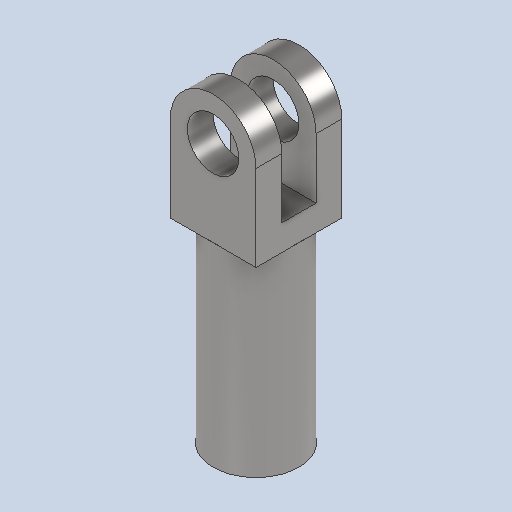
# Autodesk Inventor part: Część L5
Saved by Autodesk Inventor 2022.1 (Build 261234020, 234B)
## iProperties
Created: 2022-05-02
Part Number: Część L5
Material: Stal nierdzewna 440C
Document SubType Name: Modeling
Designer: Kacper Kaczmarski
Density: 7.75 g/cm^3
Appearance: Częściowo polerowany
Mass: 19.5633 g
Surface Area: 16.5661 cm^2
Volume: 2.5243 cm^3
Author: Kacper Kaczmarski
Autodesk Inventor part; units mm, degrees
ref_plane "YZ Plane" through (0, 0, 0) normal (1, 0, 0) x (0, 1, 0)
ref_plane "XZ Plane" through (0, 0, 0) normal (0, 1, 0) x (-1, 0, 0)
ref_plane "XY Plane" through (0, 0, 0) normal (0, 0, 1) x (1, 0, 0)
sketch "Szkic1" plane through (0, 0, 0) normal (0, 0, 1) x (1, 0, 0)
  line L0 (0, 0) -> (-10, 0)
  line L1 (-10, 0) -> (-10, 32.68)
  line L2 (-10, 32.68) -> (0, 32.68)
  line L3 (0, 32.68) -> (0, 0)
  arc A0 (0, 32.68) -> (-10, 32.68) centre (-5, 32.68) ccw
  circle A1 centre (-5, 32.68) radius 3
  dimension "d2" = 10
  dimension "d3" = 32.68
  dimension "d4" = 6
  constraints: 8 end point, 2 centre point, 2 parallel, 2 point on circle, 2 tangent, 1 coincident, 1 horizontal, 1 perpendicular
  measures "d2" distance of L1.end L2.end
  measures "d3" distance of L0.end L1.end
  measures "d4" diameter of A1
extrude "Wyciągnięcie proste1" add sketch "Szkic1" against normal blind 10 contours L0 L1 L2 A1 L3 | L2 A1 A0
sketch "Szkic2" plane through (-10, 0, 0) normal (-1, 0, 0) x (0, 0, 1)
  line L0 (-10, 29.68) -> (0, 29.68) projected
  line L1 (-13.2063, 25.68) -> (3.6302, 25.68)
  line L2 (0, 32.68) -> (-10, 32.68) projected
  line L3 (-5, 32.68) -> (-5, 38.3797)
  line L4 (-7, 25.68) -> (-3, 25.68)
  line L5 (-3, 25.68) -> (-3, 38.3797)
  line L6 (-3, 38.3797) -> (-7, 38.3797)
  line L7 (-7, 38.3797) -> (-7, 25.68)
  point P0 (0, 0)
  dimension "d7" = 7
  dimension "d8" = 4
  constraints: 12 end point, 2 horizontal, 2 parallel, 1 midpoint, 1 perpendicular, 1 point on line, 1 vertical, 1 other
  measures "d7" distance between parallel lines of L2 L1
  measures "d8" distance of L6.end L5.end
extrude "Wyciągnięcie proste2" cut sketch "Szkic2" against normal blind 10
sketch "Szkic3" plane through (-10, 0, 0) normal (0, -1, 0) x (1, 0, 0)
  line L0 (0, -10) -> (10, -10) projected
  line L1 (5, -10) -> (5, 0)
  line L2 (0, 0) -> (10, 0) projected
  line L3 (10, 0) -> (10, -10) projected
  line L4 (10, -5) -> (0, -5)
  line L5 (0, 0) -> (0, -10) projected
  point P0 (5, -5)
  constraints: 5 midpoint, 4 end point
hole "Otwór1" at (-5, 0, -5) direction (0, 1, 0) diameter 2.459 depth 8.8 tip angle 118 thread size "M3x0.5" class "6H" standard "ISO Metric profile"
sketch "Szkic4" plane through (-10, 0, 0) normal (0, -1, 0) x (1, 0, 0)
  line L0 (10, 0) -> (10, -10) projected
  line L1 (0, 0) -> (0, -10) projected
  line L2 (10, -10) -> (0, -10)
  line L3 (0, -10) -> (0, 0)
  line L4 (0, 0) -> (10, 0)
  line L5 (10, 0) -> (10, -10)
  circle A0 centre (5, -5) radius 1.2295 projected
  circle A1 centre (5, -5) radius 5
  point P0 (0, -5)
  point P1 (5, 0)
  point P2 (10, -5)
  point P3 (5, -10)
  constraints: 8 end point, 2 parallel, 1 centre point, 1 coincident, 1 horizontal, 1 perpendicular
extrude "Wyciągnięcie proste3" cut sketch "Szkic4" against normal blind 22.68 contours L0 A1 L4 | L0 L2 A1 | A1 L1 L4 | L2 L1 A1
